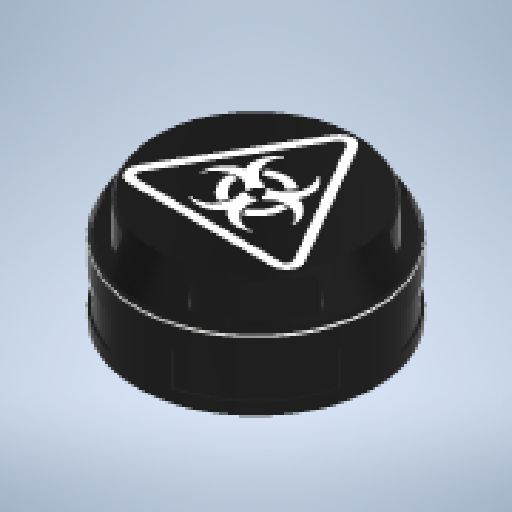
# Autodesk Inventor part: cap
Saved by Autodesk Inventor 2024.2 (Build 282272000, 272)
## iProperties
Created: 2024-09-15
Part Number: cap
Material: Plastique ABS
Document SubType Name: Modeling
Designer: Sebastien
Density: 1.06 g/cm^3
Appearance: Lisse - Noir
Author: Sebastien
Autodesk Inventor part; units mm, degrees
ref_plane "XZ Plane" through (0, 0, 0) normal (0, 1, 0) x (-1, 0, 0)
sketch "Esquisse1" plane through (0, 0, 0) normal (0, 0, 1) x (1, 0, 0)
  line L0 (43.1, 0) -> (43.1, 27.5)
  line L1 (43.1, 27.5) -> (36.1, 39.5)
  line L2 (36.1, 39.5) -> (0, 39.5)
  line L3 (0, 39.5) -> (0, 36.5)
  line L4 (0, 36.5) -> (27.6, 36.5)
  line L5 (27.6, 36.5) -> (28.15, 0)
  line L6 (43.1, 24.5) -> (27.7808, 24.5)
  line L7 (27.7658, 25.5) -> (43.1, 25.5)
  line L8 (43.1, 0) -> (41.1, 0)
  line L9 (41.1, 0) -> (41.1, 2.2)
  line L10 (28.15, 0) -> (35.9, 0)
  line L11 (35.9, 0) -> (35.9, 2.2)
  line L12 (35.9, 2.2) -> (41.1, 2.2)
  point P0 (0, 0)
  dimension "d1" = 55.2
  dimension "d2" = 56.3
  dimension "d4" = 3
  dimension "d5" = 7
  dimension "d6" = 12
  dimension "d7" = 86.2
  dimension "d20" = 1
  dimension "d21" = 2
  dimension "d23" = 2
  dimension "d24" = 2.2
  dimension "d25" = 5.2
  dimension "d26" = 39.5
  dimension "d54" = 36.5
  dimension "d55" = 0.863
  constraints: 26 end point, 6 perpendicular, 4 point on line, 3 horizontal, 2 horizontal alignment, 2 vertical, 1 vertical alignment
  measures "d1" diameter of L4.end L3
  measures "d2" diameter of L5.end L3
  measures "d4" distance of L2.end L3.end
  measures "d5" horizontal distance of L0.end L1.end
  measures "d6" vertical distance of L0.end L1.end
  measures "d7" diameter of L0 L3
  measures "d20" distance between parallel lines of L6 L7
  measures "d21" distance from line of L0.end L7
  measures "d23" distance of L0.start L8.end
  measures "d24" distance of L8.end L9.end
  measures "d25" distance of L11.end L9.end
  measures "d26" distance between parallel lines of L10 L2
  measures "d54" distance between parallel lines of L10 L4
  measures "d55" angle of L3 L5
revolve "Révolution1" add sketch "Esquisse1" angle 360 about axis through (0, 39.5, 0) along (0, -1, 0) contours L8 L9 L12 L11 L10 L5 L6 L0 | L7 L5 L4 L3 L2 L1 L0
revolve "Révolution3" add sketch "Esquisse1" angle 360 about axis through (0, 39.5, 0) along (0, -1, 0) separate body contours L6 L5 L7 L0
ref_plane "Plan de construction1" through (0, 26.5, 0) normal (0, 1, 0) x (1, 0, 0)
sketch "Esquisse2" plane through (0, 26.5, 0) normal (0, 1, 0) x (1, 0, 0)
  circle A0 centre (0, 0) radius 43.1 construction
  circle A1 centre (0, 0) radius 27.7507 construction
  arc A2 (34.2759, 14.1976) -> (14.1976, 34.2759) centre (0, 0) ccw
  arc A3 (13.0784, 36.7935) -> (14.1976, 34.2759) centre (14.9629, 36.1237) ccw
  line L0 (13.0784, 36.7935) -> (13.4138, 37.737)
  arc A4 (16.0613, 38.9159) -> (13.4138, 37.737) centre (15.2983, 37.0671) ccw
  arc A5 (38.9159, 16.0613) -> (16.0613, 38.9159) centre (0, 0) ccw
  arc A6 (37.737, 13.4138) -> (38.9159, 16.0613) centre (37.0671, 15.2983) ccw
  line L1 (37.737, 13.4138) -> (36.7935, 13.0784)
  arc A7 (34.2759, 14.1976) -> (36.7935, 13.0784) centre (36.1237, 14.9629) ccw
  circle A8 centre (0, 0) radius 36.1 construction
  line L2 (0, 0) -> (0, 62.2569) construction
  point P0 (0, 0)
  point P1 (26.2337, 26.2337)
  dimension "d28" = 2
  dimension "d29" = 1
  dimension "d30" = 1
  dimension "d31" = 45
  dimension "d37" = 45
  constraints: 13 point on circle, 8 tangent, 6 centre point, 6 end point, 3 equal radius, 2 point on line, 1 coincident, 1 concentric, 1 vertical
  measures "d28" radius of A7
  measures "d29" radial gap between concentric circles of A8 A2
  measures "d30" radial gap between concentric circles of A0 A5
extrude "Extrusion1" cut sketch "Esquisse2" along normal through all bodies 1
ref_plane "Plan de construction2" through (0, 0, 0) normal (0.7071, 0, -0.7071) x (0, 1, 0)
sketch "Esquisse3" plane through (0, 0, 0) normal (0.7071, 0, -0.7071) x (0, 1, 0)
  line L0 (27.5, 43.1) -> (27.5, -43.1) construction
  line L1 (0, 43.1) -> (0, -43.1) construction
  line L2 (24.5, 43.1) -> (0, 43.1) construction
  line L3 (16.5, 43.1) -> (4.5, 43.1)
  line L4 (4.5, 43.1) -> (4.5, 42.1)
  line L5 (4.5, 42.1) -> (16.5, 42.1)
  line L6 (16.5, 42.1) -> (16.5, 43.1)
  line L7 (0, -60.34) -> (0, 60.34) projected
  line L8 (-5.5, 0) -> (33, 0) projected
  point P0 (0, 0)
  point P1 (10.5, 43.1)
  dimension "d39" = 12
  dimension "d40" = 1
  dimension "d41" = 17
  constraints: 8 end point, 2 parallel, 1 horizontal, 1 midpoint, 1 perpendicular, 1 point on line
  measures "d39" distance of L4.end L5.end
  measures "d40" distance of L5.end L3.start
  measures "d41" distance from line of L0 point (10.5, 43.1)
revolve "Révolution4" cut sketch "Esquisse3" angle 60 mid plane about axis through (0, -10, 0) along (0, 1, 0) bodies 1
pattern_circular "Réseau circulaire2" count 4 over 360 about axis through (0, -10, 0) along (0, 1, 0) of "Extrusion1", "Révolution4" bodies 1
sketch "Esquisse4" plane through (0, 39.5, 0) normal (0, 1, 0) x (1, 0, 0)
  line L0 (-40, 41.2) -> (40, 41.2) construction
  line L1 (40, 41.2) -> (40, -38.8) construction
  line L2 (40, -38.8) -> (-40, -38.8) construction
  line L3 (-40, -38.8) -> (-40, 41.2) construction
  line L4 (-30.3109, -12.5) -> (-4.3301, 32.5)
  arc A0 (4.3301, 32.5) -> (-4.3301, 32.5) centre (0, 30) ccw
  line L5 (4.3301, 32.5) -> (30.3109, -12.5)
  arc A1 (25.9808, -20) -> (30.3109, -12.5) centre (25.9808, -15) ccw
  line L6 (25.9808, -20) -> (-25.9808, -20)
  arc A2 (-30.3109, -12.5) -> (-25.9808, -20) centre (-25.9808, -15) ccw
  line L7 (-1.7321, 31) -> (-27.7128, -14)
  arc A3 (-27.7128, -14) -> (-25.9808, -17) centre (-25.9808, -15) ccw
  line L8 (-25.9808, -17) -> (25.9808, -17)
  arc A4 (25.9808, -17) -> (27.7128, -14) centre (25.9808, -15) ccw
  line L9 (27.7128, -14) -> (1.7321, 31)
  arc A5 (1.7321, 31) -> (-1.7321, 31) centre (0, 30) ccw
  circle A6 centre (0, 0) radius 17 construction
  circle A7 centre (0, 0) radius 35 construction
  spline S0 degree 2 poles (-2.2488, 0.3977) (-2.2488, 0.0817) (-2.1029, -0.2587) knots 0 0 0 1 1 1
  line L10 (-2.1029, -0.2587) -> (-3.2212, -0.8908)
  spline S1 degree 2 poles (-3.2212, -0.8908) (-5.1661, 1.6862) (-8.3752, 1.8564) knots 0 0 0 1 1 1
  spline S2 degree 2 poles (-8.3752, 1.8564) (-11.2925, 2.0023) (-13.3833, 0.5436) knots 0 0 0 1 1 1
  spline S3 degree 2 poles (-13.3833, 0.5436) (-15.7901, -1.0609) (-16.2763, -3.1517) knots 0 0 0 1 1 1
  spline S4 degree 2 poles (-16.2763, -3.1517) (-16.2763, -3.4677) (-16.4465, -3.4677) knots 0 0 0 1 1 1
  spline S5 degree 2 poles (-16.4465, -3.4677) (-16.9327, -3.4677) (-16.7626, -2.4953) knots 0 0 0 1 1 1
  spline S6 degree 2 poles (-16.7626, -2.4953) (-16.5924, -0.7449) (-15.6199, 1.0298) knots 0 0 0 1 1 1
  spline S7 degree 2 poles (-15.6199, 1.0298) (-14.5016, 3.1449) (-12.8971, 4.2632) knots 0 0 0 1 1 1
  spline S8 degree 2 poles (-12.8971, 4.2632) (-10.9522, 5.5517) (-9.5178, 5.5517) knots 0 0 0 1 1 1
  spline S9 degree 2 poles (-9.5178, 5.5517) (-9.5178, 5.8677) (-9.9797, 7.1562) knots 0 0 0 1 1 1
  spline S10 degree 2 poles (-9.9797, 7.1562) (-10.3201, 8.2989) (-10.3201, 9.1011) knots 0 0 0 1 1 1
  spline S11 degree 2 poles (-10.3201, 9.1011) (-10.3201, 13.1368) (-6.7707, 16.3459) knots 0 0 0 1 1 1
  spline S12 degree 2 poles (-6.7707, 16.3459) (-6.4546, 16.516) (-6.2844, 16.516) knots 0 0 0 1 1 1
  spline S13 degree 2 poles (-6.2844, 16.516) (-5.9684, 16.516) (-5.9684, 16.3459) knots 0 0 0 1 1 1
  spline S14 degree 2 poles (-5.9684, 16.3459) (-5.9684, 16.2) (-6.1143, 16.0298) knots 0 0 0 1 1 1
  spline S15 degree 2 poles (-6.1143, 16.0298) (-7.5729, 14.4253) (-7.5729, 11.5079) knots 0 0 0 1 1 1
  spline S16 degree 2 poles (-7.5729, 11.5079) (-7.4028, 8.4447) (-5.4822, 6.354) knots 0 0 0 1 1 1
  spline S17 degree 2 poles (-5.4822, 6.354) (-3.3914, 4.093) (-0.6442, 3.9472) knots 0 0 0 1 1 1
  line L11 (-0.6442, 3.9472) -> (-0.6442, 2.4885)
  spline S18 degree 2 poles (-0.6442, 2.4885) (-2.2488, 2.0023) (-2.2488, 0.3977) knots 0 0 0 1 1 1
  spline S19 degree 2 poles (2.1029, -0.2587) (2.2488, 0.0817) (2.2488, 0.3977) knots 0 0 0 1 1 1
  spline S20 degree 2 poles (2.2488, 0.3977) (2.419, 2.0023) (0.6442, 2.4885) knots 0 0 0 1 1 1
  line L12 (0.6442, 2.4885) -> (0.6442, 3.9472)
  spline S21 degree 2 poles (0.6442, 3.9472) (3.5373, 4.093) (5.4822, 6.354) knots 0 0 0 1 1 1
  spline S22 degree 2 poles (5.4822, 6.354) (7.5729, 8.4447) (7.5729, 11.5079) knots 0 0 0 1 1 1
  spline S23 degree 2 poles (7.5729, 11.5079) (7.5729, 14.4253) (6.1143, 16.0298) knots 0 0 0 1 1 1
  spline S24 degree 2 poles (6.1143, 16.0298) (5.9684, 16.2) (5.9684, 16.3459) knots 0 0 0 1 1 1
  spline S25 degree 2 poles (5.9684, 16.3459) (5.9684, 16.516) (6.2844, 16.516) knots 0 0 0 1 1 1
  spline S26 degree 2 poles (6.2844, 16.516) (6.6005, 16.516) (6.7707, 16.3459) knots 0 0 0 1 1 1
  spline S27 degree 2 poles (6.7707, 16.3459) (10.466, 13.2827) (10.3201, 9.1011) knots 0 0 0 1 1 1
  spline S28 degree 2 poles (10.3201, 9.1011) (10.3201, 8.2989) (9.8339, 7.0104) knots 0 0 0 1 1 1
  spline S29 degree 2 poles (9.8339, 7.0104) (9.5178, 6.0379) (9.5178, 5.5517) knots 0 0 0 1 1 1
  spline S30 degree 2 poles (9.5178, 5.5517) (10.9522, 5.5517) (12.8971, 4.2632) knots 0 0 0 1 1 1
  spline S31 degree 2 poles (12.8971, 4.2632) (14.5016, 3.1449) (15.4741, 1.2) knots 0 0 0 1 1 1
  spline S32 degree 2 poles (15.4741, 1.2) (16.5924, -0.7449) (16.7626, -2.6655) knots 0 0 0 1 1 1
  spline S33 degree 2 poles (16.7626, -2.6655) (16.7626, -3.4677) (16.4465, -3.4677) knots 0 0 0 1 1 1
  spline S34 degree 2 poles (16.4465, -3.4677) (16.2763, -3.4677) (16.2763, -3.1517) knots 0 0 0 1 1 1
  spline S35 degree 2 poles (16.2763, -3.1517) (15.7901, -1.0609) (13.5292, 0.3977) knots 0 0 0 1 1 1
  spline S36 degree 2 poles (13.5292, 0.3977) (10.9522, 2.1724) (8.2293, 1.8564) knots 0 0 0 1 1 1
  spline S37 degree 2 poles (8.2293, 1.8564) (5.1661, 1.516) (3.2212, -0.8908) knots 0 0 0 1 1 1
  line L13 (3.2212, -0.8908) -> (2.1029, -0.2587)
  spline S38 degree 2 poles (0.0122, -2.1793) (0.9603, -2.3494) (1.6167, -1.5472) knots 0 0 0 1 1 1
  line L14 (1.6167, -1.5472) -> (2.5891, -2.1793)
  spline S39 degree 2 poles (2.5891, -2.1793) (2.1029, -3.6379) (2.1029, -5.2425) knots 0 0 0 1 1 1
  spline S40 degree 2 poles (2.1029, -5.2425) (2.2488, -7.3332) (3.2212, -8.9621) knots 0 0 0 1 1 1
  spline S41 degree 2 poles (3.2212, -8.9621) (4.3395, -10.7368) (6.2844, -11.6849) knots 0 0 0 1 1 1
  spline S42 degree 2 poles (6.2844, -11.6849) (8.0592, -12.6574) (9.6637, -12.6574) knots 0 0 0 1 1 1
  spline S43 degree 2 poles (9.6637, -12.6574) (10.1499, -12.6574) (10.3201, -12.4872) knots 0 0 0 1 1 1
  spline S44 degree 2 poles (10.3201, -12.4872) (10.9522, -12.4872) (11.1224, -12.4872) knots 0 0 0 1 1 1
  spline S45 degree 2 poles (11.1224, -12.4872) (11.4384, -12.9734) (10.9522, -13.1436) knots 0 0 0 1 1 1
  spline S46 degree 2 poles (10.9522, -13.1436) (8.8614, -13.9459) (6.7707, -13.9459) knots 0 0 0 1 1 1
  spline S47 degree 2 poles (6.7707, -13.9459) (4.6799, -13.9459) (2.9052, -12.9734) knots 0 0 0 1 1 1
  spline S48 degree 2 poles (2.9052, -12.9734) (0.8144, -11.8551) (0.0122, -10.7368) knots 0 0 0 1 1 1
  spline S49 degree 2 poles (0.0122, -10.7368) (-0.3282, -10.8827) (-1.1305, -11.8551) knots 0 0 0 1 1 1
  spline S50 degree 2 poles (-1.1305, -11.8551) (-1.7626, -12.6574) (-2.419, -12.9734) knots 0 0 0 1 1 1
  spline S51 degree 2 poles (-2.419, -12.9734) (-4.1937, -14.116) (-6.6005, -14.116) knots 0 0 0 1 1 1
  spline S52 degree 2 poles (-6.6005, -14.116) (-9.0316, -14.116) (-10.8063, -13.4596) knots 0 0 0 1 1 1
  spline S53 degree 2 poles (-10.8063, -13.4596) (-11.1224, -13.3138) (-11.1224, -12.9734) knots 0 0 0 1 1 1
  spline S54 degree 2 poles (-11.1224, -12.9734) (-11.1224, -12.8276) (-10.9522, -12.8276) knots 0 0 0 1 1 1
  spline S55 degree 2 poles (-10.9522, -12.8276) (-10.8063, -12.8276) (-10.3201, -12.8276) knots 0 0 0 1 1 1
  spline S56 degree 2 poles (-10.3201, -12.8276) (-9.8339, -12.9734) (-9.6637, -12.9734) knots 0 0 0 1 1 1
  spline S57 degree 2 poles (-9.6637, -12.9734) (-7.889, -12.9734) (-6.1143, -12.0253) knots 0 0 0 1 1 1
  spline S58 degree 2 poles (-6.1143, -12.0253) (-4.3395, -11.1987) (-3.3914, -9.2781) knots 0 0 0 1 1 1
  spline S59 degree 2 poles (-3.3914, -9.2781) (-2.2488, -7.3332) (-2.2488, -5.5585) knots 0 0 0 1 1 1
  spline S60 degree 2 poles (-2.2488, -5.5585) (-2.2488, -3.7838) (-2.9052, -2.1793) knots 0 0 0 1 1 1
  line L15 (-2.9052, -2.1793) -> (-1.6167, -1.5472)
  spline S61 degree 2 poles (-1.6167, -1.5472) (-0.9603, -2.1793) (0.0122, -2.1793) knots 0 0 0 1 1 1
  spline S62 degree 2 poles (-3.2212, -6.531) (-3.3914, -8.1355) (-4.3395, -9.2781) knots 0 0 0 1 1 1
  spline S63 degree 2 poles (-4.3395, -9.2781) (-7.2569, -8.1355) (-9.0316, -5.0966) knots 0 0 0 1 1 1
  spline S64 degree 2 poles (-9.0316, -5.0966) (-10.6361, -2.6655) (-10.6361, 0.3977) knots 0 0 0 1 1 1
  spline S65 degree 2 poles (-10.6361, 0.3977) (-10.466, 0.884) (-10.466, 1.2) knots 0 0 0 1 1 1
  spline S66 degree 2 poles (-10.466, 1.2) (-9.8339, 1.2) (-9.5178, 1.2) knots 0 0 0 1 1 1
  spline S67 degree 2 poles (-9.5178, 1.2) (-8.3752, 1.2) (-7.5729, 0.884) knots 0 0 0 1 1 1
  spline S68 degree 2 poles (-7.5729, 0.884) (-7.5729, 0.5436) (-7.5729, 0.3977) knots 0 0 0 1 1 1
  spline S69 degree 2 poles (-7.5729, 0.3977) (-7.5729, -1.693) (-6.6005, -3.3219) knots 0 0 0 1 1 1
  spline S70 degree 2 poles (-6.6005, -3.3219) (-5.312, -5.5585) (-3.2212, -6.531) knots 0 0 0 1 1 1
  spline S71 degree 2 poles (9.0316, -5.0966) (7.4028, -7.9896) (4.3395, -9.2781) knots 0 0 0 1 1 1
  spline S72 degree 2 poles (4.3395, -9.2781) (3.5373, -8.1355) (3.2212, -6.531) knots 0 0 0 1 1 1
  spline S73 degree 2 poles (3.2212, -6.531) (5.312, -5.5585) (6.4546, -3.4677) knots 0 0 0 1 1 1
  spline S74 degree 2 poles (6.4546, -3.4677) (7.5729, -1.693) (7.5729, 0.3977) knots 0 0 0 1 1 1
  spline S75 degree 2 poles (7.5729, 0.3977) (7.5729, 0.7138) (7.5729, 0.884) knots 0 0 0 1 1 1
  spline S76 degree 2 poles (7.5729, 0.884) (8.3752, 1.2) (9.5178, 1.2) knots 0 0 0 1 1 1
  spline S77 degree 2 poles (9.5178, 1.2) (10.1499, 1.2) (10.6361, 1.2) knots 0 0 0 1 1 1
  spline S78 degree 2 poles (10.6361, 1.2) (10.8063, 0.884) (10.466, -0.2587) knots 0 0 0 1 1 1
  spline S79 degree 2 poles (10.466, -0.2587) (10.3201, -2.9815) (9.0316, -5.0966) knots 0 0 0 1 1 1
  spline S80 degree 2 poles (0.0122, 11.0217) (3.3914, 11.0217) (5.9684, 9.1011) knots 0 0 0 1 1 1
  spline S81 degree 2 poles (5.9684, 9.1011) (5.312, 7.6425) (4.1937, 6.67) knots 0 0 0 1 1 1
  spline S82 degree 2 poles (4.1937, 6.67) (2.419, 7.9585) (0.3282, 7.9585) knots 0 0 0 1 1 1
  spline S83 degree 2 poles (0.3282, 7.9585) (-2.1029, 7.9585) (-4.1937, 6.67) knots 0 0 0 1 1 1
  spline S84 degree 2 poles (-4.1937, 6.67) (-5.1661, 7.4966) (-5.9684, 9.1011) knots 0 0 0 1 1 1
  spline S85 degree 2 poles (-5.9684, 9.1011) (-3.0511, 11.0217) (0.0122, 11.0217) knots 0 0 0 1 1 1
  spline S86 degree 2 poles (-2.2488, 0.3977) (-2.2488, 0.0817) (-2.1029, -0.2587) knots 0 0 0 1 1 1
  line L16 (-2.1029, -0.2587) -> (-3.2212, -0.8908)
  spline S87 degree 2 poles (-3.2212, -0.8908) (-5.1661, 1.6862) (-8.3752, 1.8564) knots 0 0 0 1 1 1
  spline S88 degree 2 poles (-8.3752, 1.8564) (-11.2925, 2.0023) (-13.3833, 0.5436) knots 0 0 0 1 1 1
  spline S89 degree 2 poles (-13.3833, 0.5436) (-15.7901, -1.0609) (-16.2763, -3.1517) knots 0 0 0 1 1 1
  spline S90 degree 2 poles (-16.2763, -3.1517) (-16.2763, -3.4677) (-16.4465, -3.4677) knots 0 0 0 1 1 1
  spline S91 degree 2 poles (-16.4465, -3.4677) (-16.9327, -3.4677) (-16.7626, -2.4953) knots 0 0 0 1 1 1
  spline S92 degree 2 poles (-16.7626, -2.4953) (-16.5924, -0.7449) (-15.6199, 1.0298) knots 0 0 0 1 1 1
  spline S93 degree 2 poles (-15.6199, 1.0298) (-14.5016, 3.1449) (-12.8971, 4.2632) knots 0 0 0 1 1 1
  spline S94 degree 2 poles (-12.8971, 4.2632) (-10.9522, 5.5517) (-9.5178, 5.5517) knots 0 0 0 1 1 1
  spline S95 degree 2 poles (-9.5178, 5.5517) (-9.5178, 5.8677) (-9.9797, 7.1562) knots 0 0 0 1 1 1
  spline S96 degree 2 poles (-9.9797, 7.1562) (-10.3201, 8.2989) (-10.3201, 9.1011) knots 0 0 0 1 1 1
  spline S97 degree 2 poles (-10.3201, 9.1011) (-10.3201, 13.1368) (-6.7707, 16.3459) knots 0 0 0 1 1 1
  spline S98 degree 2 poles (-6.7707, 16.3459) (-6.4546, 16.516) (-6.2844, 16.516) knots 0 0 0 1 1 1
  spline S99 degree 2 poles (-6.2844, 16.516) (-5.9684, 16.516) (-5.9684, 16.3459) knots 0 0 0 1 1 1
  spline S100 degree 2 poles (-5.9684, 16.3459) (-5.9684, 16.2) (-6.1143, 16.0298) knots 0 0 0 1 1 1
  spline S101 degree 2 poles (-6.1143, 16.0298) (-7.5729, 14.4253) (-7.5729, 11.5079) knots 0 0 0 1 1 1
  spline S102 degree 2 poles (-7.5729, 11.5079) (-7.4028, 8.4447) (-5.4822, 6.354) knots 0 0 0 1 1 1
  spline S103 degree 2 poles (-5.4822, 6.354) (-3.3914, 4.093) (-0.6442, 3.9472) knots 0 0 0 1 1 1
  line L17 (-0.6442, 3.9472) -> (-0.6442, 2.4885)
  spline S104 degree 2 poles (-0.6442, 2.4885) (-2.2488, 2.0023) (-2.2488, 0.3977) knots 0 0 0 1 1 1
  spline S105 degree 2 poles (2.1029, -0.2587) (2.2488, 0.0817) (2.2488, 0.3977) knots 0 0 0 1 1 1
  spline S106 degree 2 poles (2.2488, 0.3977) (2.419, 2.0023) (0.6442, 2.4885) knots 0 0 0 1 1 1
  line L18 (0.6442, 2.4885) -> (0.6442, 3.9472)
  spline S107 degree 2 poles (0.6442, 3.9472) (3.5373, 4.093) (5.4822, 6.354) knots 0 0 0 1 1 1
  spline S108 degree 2 poles (5.4822, 6.354) (7.5729, 8.4447) (7.5729, 11.5079) knots 0 0 0 1 1 1
  spline S109 degree 2 poles (7.5729, 11.5079) (7.5729, 14.4253) (6.1143, 16.0298) knots 0 0 0 1 1 1
  spline S110 degree 2 poles (6.1143, 16.0298) (5.9684, 16.2) (5.9684, 16.3459) knots 0 0 0 1 1 1
  spline S111 degree 2 poles (5.9684, 16.3459) (5.9684, 16.516) (6.2844, 16.516) knots 0 0 0 1 1 1
  spline S112 degree 2 poles (6.2844, 16.516) (6.6005, 16.516) (6.7707, 16.3459) knots 0 0 0 1 1 1
  spline S113 degree 2 poles (6.7707, 16.3459) (10.466, 13.2827) (10.3201, 9.1011) knots 0 0 0 1 1 1
  spline S114 degree 2 poles (10.3201, 9.1011) (10.3201, 8.2989) (9.8339, 7.0104) knots 0 0 0 1 1 1
  spline S115 degree 2 poles (9.8339, 7.0104) (9.5178, 6.0379) (9.5178, 5.5517) knots 0 0 0 1 1 1
  spline S116 degree 2 poles (9.5178, 5.5517) (10.9522, 5.5517) (12.8971, 4.2632) knots 0 0 0 1 1 1
  spline S117 degree 2 poles (12.8971, 4.2632) (14.5016, 3.1449) (15.4741, 1.2) knots 0 0 0 1 1 1
  spline S118 degree 2 poles (15.4741, 1.2) (16.5924, -0.7449) (16.7626, -2.6655) knots 0 0 0 1 1 1
  spline S119 degree 2 poles (16.7626, -2.6655) (16.7626, -3.4677) (16.4465, -3.4677) knots 0 0 0 1 1 1
  spline S120 degree 2 poles (16.4465, -3.4677) (16.2763, -3.4677) (16.2763, -3.1517) knots 0 0 0 1 1 1
  spline S121 degree 2 poles (16.2763, -3.1517) (15.7901, -1.0609) (13.5292, 0.3977) knots 0 0 0 1 1 1
  spline S122 degree 2 poles (13.5292, 0.3977) (10.9522, 2.1724) (8.2293, 1.8564) knots 0 0 0 1 1 1
  spline S123 degree 2 poles (8.2293, 1.8564) (5.1661, 1.516) (3.2212, -0.8908) knots 0 0 0 1 1 1
  line L19 (3.2212, -0.8908) -> (2.1029, -0.2587)
  spline S124 degree 2 poles (0.0122, -2.1793) (0.9603, -2.3494) (1.6167, -1.5472) knots 0 0 0 1 1 1
  line L20 (1.6167, -1.5472) -> (2.5891, -2.1793)
  spline S125 degree 2 poles (2.5891, -2.1793) (2.1029, -3.6379) (2.1029, -5.2425) knots 0 0 0 1 1 1
  spline S126 degree 2 poles (2.1029, -5.2425) (2.2488, -7.3332) (3.2212, -8.9621) knots 0 0 0 1 1 1
  spline S127 degree 2 poles (3.2212, -8.9621) (4.3395, -10.7368) (6.2844, -11.6849) knots 0 0 0 1 1 1
  spline S128 degree 2 poles (6.2844, -11.6849) (8.0592, -12.6574) (9.6637, -12.6574) knots 0 0 0 1 1 1
  spline S129 degree 2 poles (9.6637, -12.6574) (10.1499, -12.6574) (10.3201, -12.4872) knots 0 0 0 1 1 1
  spline S130 degree 2 poles (10.3201, -12.4872) (10.9522, -12.4872) (11.1224, -12.4872) knots 0 0 0 1 1 1
  spline S131 degree 2 poles (11.1224, -12.4872) (11.4384, -12.9734) (10.9522, -13.1436) knots 0 0 0 1 1 1
  spline S132 degree 2 poles (10.9522, -13.1436) (8.8614, -13.9459) (6.7707, -13.9459) knots 0 0 0 1 1 1
  spline S133 degree 2 poles (6.7707, -13.9459) (4.6799, -13.9459) (2.9052, -12.9734) knots 0 0 0 1 1 1
  spline S134 degree 2 poles (2.9052, -12.9734) (0.8144, -11.8551) (0.0122, -10.7368) knots 0 0 0 1 1 1
  spline S135 degree 2 poles (0.0122, -10.7368) (-0.3282, -10.8827) (-1.1305, -11.8551) knots 0 0 0 1 1 1
  spline S136 degree 2 poles (-1.1305, -11.8551) (-1.7626, -12.6574) (-2.419, -12.9734) knots 0 0 0 1 1 1
  spline S137 degree 2 poles (-2.419, -12.9734) (-4.1937, -14.116) (-6.6005, -14.116) knots 0 0 0 1 1 1
  spline S138 degree 2 poles (-6.6005, -14.116) (-9.0316, -14.116) (-10.8063, -13.4596) knots 0 0 0 1 1 1
  spline S139 degree 2 poles (-10.8063, -13.4596) (-11.1224, -13.3138) (-11.1224, -12.9734) knots 0 0 0 1 1 1
  spline S140 degree 2 poles (-11.1224, -12.9734) (-11.1224, -12.8276) (-10.9522, -12.8276) knots 0 0 0 1 1 1
  spline S141 degree 2 poles (-10.9522, -12.8276) (-10.8063, -12.8276) (-10.3201, -12.8276) knots 0 0 0 1 1 1
  spline S142 degree 2 poles (-10.3201, -12.8276) (-9.8339, -12.9734) (-9.6637, -12.9734) knots 0 0 0 1 1 1
  spline S143 degree 2 poles (-9.6637, -12.9734) (-7.889, -12.9734) (-6.1143, -12.0253) knots 0 0 0 1 1 1
  spline S144 degree 2 poles (-6.1143, -12.0253) (-4.3395, -11.1987) (-3.3914, -9.2781) knots 0 0 0 1 1 1
  spline S145 degree 2 poles (-3.3914, -9.2781) (-2.2488, -7.3332) (-2.2488, -5.5585) knots 0 0 0 1 1 1
  spline S146 degree 2 poles (-2.2488, -5.5585) (-2.2488, -3.7838) (-2.9052, -2.1793) knots 0 0 0 1 1 1
  line L21 (-2.9052, -2.1793) -> (-1.6167, -1.5472)
  spline S147 degree 2 poles (-1.6167, -1.5472) (-0.9603, -2.1793) (0.0122, -2.1793) knots 0 0 0 1 1 1
  spline S148 degree 2 poles (-3.2212, -6.531) (-3.3914, -8.1355) (-4.3395, -9.2781) knots 0 0 0 1 1 1
  spline S149 degree 2 poles (-4.3395, -9.2781) (-7.2569, -8.1355) (-9.0316, -5.0966) knots 0 0 0 1 1 1
  spline S150 degree 2 poles (-9.0316, -5.0966) (-10.6361, -2.6655) (-10.6361, 0.3977) knots 0 0 0 1 1 1
  spline S151 degree 2 poles (-10.6361, 0.3977) (-10.466, 0.884) (-10.466, 1.2) knots 0 0 0 1 1 1
  spline S152 degree 2 poles (-10.466, 1.2) (-9.8339, 1.2) (-9.5178, 1.2) knots 0 0 0 1 1 1
  spline S153 degree 2 poles (-9.5178, 1.2) (-8.3752, 1.2) (-7.5729, 0.884) knots 0 0 0 1 1 1
  spline S154 degree 2 poles (-7.5729, 0.884) (-7.5729, 0.5436) (-7.5729, 0.3977) knots 0 0 0 1 1 1
  spline S155 degree 2 poles (-7.5729, 0.3977) (-7.5729, -1.693) (-6.6005, -3.3219) knots 0 0 0 1 1 1
  spline S156 degree 2 poles (-6.6005, -3.3219) (-5.312, -5.5585) (-3.2212, -6.531) knots 0 0 0 1 1 1
  spline S157 degree 2 poles (9.0316, -5.0966) (7.4028, -7.9896) (4.3395, -9.2781) knots 0 0 0 1 1 1
  spline S158 degree 2 poles (4.3395, -9.2781) (3.5373, -8.1355) (3.2212, -6.531) knots 0 0 0 1 1 1
  spline S159 degree 2 poles (3.2212, -6.531) (5.312, -5.5585) (6.4546, -3.4677) knots 0 0 0 1 1 1
  spline S160 degree 2 poles (6.4546, -3.4677) (7.5729, -1.693) (7.5729, 0.3977) knots 0 0 0 1 1 1
  spline S161 degree 2 poles (7.5729, 0.3977) (7.5729, 0.7138) (7.5729, 0.884) knots 0 0 0 1 1 1
  spline S162 degree 2 poles (7.5729, 0.884) (8.3752, 1.2) (9.5178, 1.2) knots 0 0 0 1 1 1
  spline S163 degree 2 poles (9.5178, 1.2) (10.1499, 1.2) (10.6361, 1.2) knots 0 0 0 1 1 1
  spline S164 degree 2 poles (10.6361, 1.2) (10.8063, 0.884) (10.466, -0.2587) knots 0 0 0 1 1 1
  spline S165 degree 2 poles (10.466, -0.2587) (10.3201, -2.9815) (9.0316, -5.0966) knots 0 0 0 1 1 1
  spline S166 degree 2 poles (0.0122, 11.0217) (3.3914, 11.0217) (5.9684, 9.1011) knots 0 0 0 1 1 1
  spline S167 degree 2 poles (5.9684, 9.1011) (5.312, 7.6425) (4.1937, 6.67) knots 0 0 0 1 1 1
  spline S168 degree 2 poles (4.1937, 6.67) (2.419, 7.9585) (0.3282, 7.9585) knots 0 0 0 1 1 1
  spline S169 degree 2 poles (0.3282, 7.9585) (-2.1029, 7.9585) (-4.1937, 6.67) knots 0 0 0 1 1 1
  spline S170 degree 2 poles (-4.1937, 6.67) (-5.1661, 7.4966) (-5.9684, 9.1011) knots 0 0 0 1 1 1
  spline S171 degree 2 poles (-5.9684, 9.1011) (-3.0511, 11.0217) (0.0122, 11.0217) knots 0 0 0 1 1 1
  point P0 (0, 0)
  point P1 (-40, 1.2)
  point P2 (0, 41.2)
  point P3 (0, 32)
  point P4 (27.7128, -16)
  point P5 (-27.7128, -16)
  dimension "d43" = 80
  dimension "d44" = 1.2
  dimension "d49" = 3
  dimension "d50" = 5
  dimension "d51" = 70
  constraints: 12 end point, 12 point on circle, 10 tangent, 8 centre point, 3 equal length, 2 coincident, 2 equal radius, 2 horizontal, 2 midpoint, 1 vertical alignment, 7 other
  measures "d43" distance of L0.start L0.end
  measures "d44" vertical distance of point (0, 0) point (-40, 1.2)
  measures "d49" distance between parallel lines of L4 L7
  measures "d50" radius of A0
  measures "d51" diameter of A7
extrude "Extrusion2" cut sketch "Esquisse4" against normal blind 0.6 contours L4 A0 L5 A1 L6 A2 bodies 1
extrude "Extrusion4" cut sketch "Esquisse4" against normal up to surface (3 mm away) contours S0 L10 S1 S2 S3 S4 S5 S6 S7 S8 S9 S10 S11 S12 S13 S14 S15 S16 S17 L11 S18 | S19 S20 L12 S21 S22 S23 S24 S25 S26 S27 S28 S29 S30 S31 S32 S33 S34 S35 S36 S37 L13 | S38 L14 S39 S40 S41 S42 S43 S44 S45 S46 S47 S48 S49 S50 S51 S52 S53 S54 S55 S56 S57 S58 S59 S60 L15 S61 | S62 S63 S64 S65 S66 S67 S68 S69 S70 | S71 S72 S73 S74 S75 S76 S77 S78 S79 | S80 S81 S82 S83 S84 S85 bodies 1
extrude "Extrusion3" add sketch "Esquisse4" against normal blind 0.6 separate body
